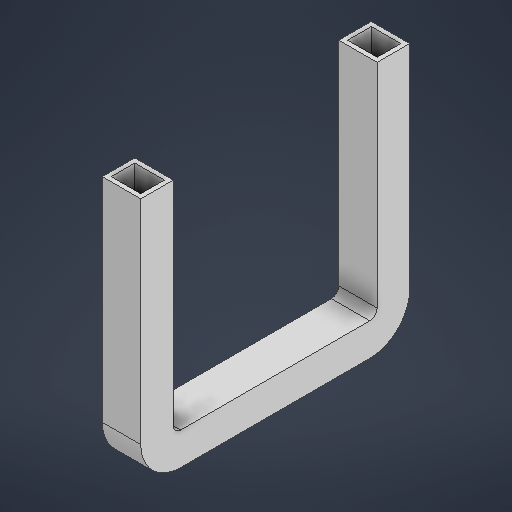
# Autodesk Inventor part: Part4
Saved by Autodesk Inventor 2026 (Build 300175050, 175E)
## iProperties
Created: 2026-04-23
Part Number: Part4
Material: Generic
Document SubType Name: Modeling
Designer: Administrator
Density: 1 g/cm^3
Appearance: Default
Author: Administrator
Autodesk Inventor part; units mm, degrees
ref_plane "YZ Plane" through (0, 0, 0) normal (1, 0, 0) x (0, 1, 0)
ref_plane "XZ Plane" through (0, 0, 0) normal (0, 1, 0) x (-1, 0, 0)
ref_plane "XY Plane" through (0, 0, 0) normal (0, 0, 1) x (1, 0, 0)
sketch "Sketch1" plane through (0, 0, 0) normal (1, 0, 0) x (0, 1, 0)
  line L0 (0, 0) -> (-72, 0)
  line L1 (-80, -8) -> (-80, -72)
  line L2 (-72, -80) -> (0, -80)
  arc A0 (-72, 0) -> (-80, -8) centre (-72, -8) ccw
  arc A1 (-80, -72) -> (-72, -80) centre (-72, -72) ccw
  point P0 (-80, 0)
  point P1 (-80, -80)
  dimension "d0" = 80
  dimension "d1" = 80
  dimension "d2" = 80
  dimension "d3" = 8
  constraints: 6 end point, 4 point on circle, 4 point on line, 4 tangent, 2 centre point, 2 perpendicular, 1 equal radius, 1 horizontal
  measures "d0" distance of point (-80, -80) L2.end
  measures "d1" distance of point (-80, 0) point (-80, -80)
  measures "d2" distance of L0.start point (-80, 0)
  measures "d3" radius of A0
sketch "Sketch2" plane through (0, 0, 0) normal (0, 1, 0) x (-1, 0, 0)
  line L0 (5, -4) -> (-5, -4)
  line L1 (-5, -4) -> (-5, 4)
  line L2 (-5, 4) -> (5, 4)
  line L3 (5, 4) -> (5, -4)
  line L4 (5, -4) -> (-5, 4) construction
  line L5 (-5, -4) -> (5, 4) construction
  line L6 (-6.5, -5.5) -> (6.5, -5.5)
  line L7 (6.5, -5.5) -> (6.5, 5.5)
  line L8 (6.5, 5.5) -> (-6.5, 5.5)
  line L9 (-6.5, 5.5) -> (-6.5, -5.5)
  point P0 (0, 0)
  dimension "d4" = 10
  dimension "d5" = 8
  dimension "d6" = 1.5
  constraints: 20 end point, 4 parallel, 2 midpoint, 2 perpendicular, 1 horizontal, 3 other
  measures "d4" distance of L1.end L2.end
  measures "d5" distance of L0.end L1.end
  measures "d6" distance between parallel lines of L0 L6
sweep "Sweep1" add profiles "Sketch2" path "Sketch1"
body "Solid1"
